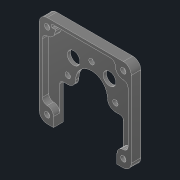
# Autodesk Inventor part: base47
Saved by Autodesk Inventor 2022 (Build 260153000, 153)
## iProperties
Created: 2021-09-10
Part Number: base47
Material: ABS プラスチック
Document SubType Name: Modeling
Designer: Yuta Kage
Density: 1.06 g/cm^3
Appearance: 滑らか - 黒
Author: Yuta Kage
Autodesk Inventor part; units mm, degrees
ref_plane "YZ Plane" through (0, 0, 0) normal (1, 0, 0) x (0, 1, 0)
ref_plane "XZ Plane" through (0, 0, 0) normal (0, 1, 0) x (-1, 0, 0)
ref_plane "XY Plane" through (0, 0, 0) normal (0, 0, 1) x (1, 0, 0)
sketch "スケッチ1" plane through (0, 0, 0) normal (0, 0, 1) x (1, 0, 0)
  line L0 (-29, -29) -> (29, -29)
  line L1 (29, -29) -> (29, 29)
  line L2 (29, 29) -> (-29, 29)
  line L3 (-29, 29) -> (-29, -29)
  line L4 (-29, -29) -> (29, 29) construction
  line L5 (29, -29) -> (-29, 29) construction
  point P0 (0, 0)
  dimension "d0" = 58
  dimension "d1" = 58
  constraints: 12 end point, 2 midpoint, 2 parallel, 1 horizontal, 1 perpendicular
  measures "d0" distance of L2.end L1.end
  measures "d1" distance of L1.end L0.end
extrude "押し出し1" add sketch "スケッチ1" along normal blind 6
fillet "フィレット1" radius 5 4 edges at (-29, 29, 3) (29, 29, 3) (29, -29, 3) (-29, -29, 3)
sketch "スケッチ4" plane through (0, 0, 6) normal (0, 0, 1) x (1, 0, 0)
  arc A0 (-29, -24) -> (-24, -29) centre (-24, -24) ccw projected
  line L0 (-24, -29) -> (24, -29) projected
  arc A1 (24, -29) -> (29, -24) centre (24, -24) ccw projected
  line L1 (29, -24) -> (29, 24) projected
  arc A2 (29, 24) -> (24, 29) centre (24, 24) ccw projected
  line L2 (24, 29) -> (-24, 29) projected
  arc A3 (-24, 29) -> (-29, 24) centre (-24, 24) ccw projected
  line L3 (-29, 24) -> (-29, -24) projected
  line L4 (-27, -27) -> (27, -27)
  line L5 (27, -27) -> (27, 27)
  line L6 (27, 27) -> (-27, 27)
  line L7 (-27, 27) -> (-27, -27)
  line L8 (-27, -27) -> (27, 27) construction
  line L9 (27, -27) -> (-27, 27) construction
  line L10 (-24, -24) -> (24, -24) construction
  line L11 (24, -24) -> (24, 24) construction
  line L12 (24, 24) -> (-24, 24) construction
  line L13 (-24, 24) -> (-24, -24) construction
  line L14 (-24, -24) -> (24, 24) construction
  line L15 (24, -24) -> (-24, 24) construction
  line L16 (24, 29) -> (-24, 29) projected
  circle A4 centre (-24, 24) radius 5
  circle A5 centre (24, 24) radius 5
  arc A6 (24, -29) -> (29, -24) centre (24, -24) ccw projected
  circle A7 centre (24, -24) radius 5
  line L17 (-24, -29) -> (24, -29) projected
  circle A8 centre (-24, -24) radius 5
  line L18 (-29, 29) -> (-19, 29)
  line L19 (-19, 29) -> (-19, 19)
  line L20 (-19, 19) -> (-29, 19)
  line L21 (-29, 19) -> (-29, 29)
  line L22 (-29, 29) -> (-19, 19) construction
  line L23 (-19, 29) -> (-29, 19) construction
  line L24 (29, 29) -> (19, 29)
  line L25 (19, 29) -> (19, 19)
  line L26 (19, 19) -> (29, 19)
  line L27 (29, 19) -> (29, 29)
  line L28 (29, 29) -> (19, 19) construction
  line L29 (19, 29) -> (29, 19) construction
  line L30 (29, -29) -> (19, -29)
  line L31 (19, -29) -> (19, -19)
  line L32 (19, -19) -> (29, -19)
  line L33 (29, -19) -> (29, -29)
  line L34 (29, -29) -> (19, -19) construction
  line L35 (19, -29) -> (29, -19) construction
  line L36 (-29, -29) -> (-19, -29)
  line L37 (-19, -29) -> (-19, -19)
  line L38 (-19, -19) -> (-29, -19)
  line L39 (-29, -19) -> (-29, -29)
  line L40 (-29, -29) -> (-19, -19) construction
  line L41 (-19, -29) -> (-29, -19) construction
  point P0 (0, 0)
  point P1 (-20, -27)
  point P2 (20, -27)
  point P3 (27, -20)
  point P4 (27, 20)
  point P5 (20, 27)
  point P6 (-20, 27)
  point P7 (-27, 20)
  point P8 (-27, -20)
  point P9 (-19, -24)
  point P10 (-19, -27)
  point P11 (19, -27)
  point P12 (19, -24)
  point P13 (24, -19)
  point P14 (27, -19)
  point P15 (27, 19)
  point P16 (24, 19)
  point P17 (19, 24)
  point P18 (19, 27)
  point P19 (-19, 27)
  point P20 (-19, 24)
  point P21 (-24, 19)
  point P22 (-27, 19)
  point P23 (-27, -19)
  point P24 (-24, -19)
  dimension "d77" = 54
  dimension "d78" = 54
  dimension "d79" = 48
  dimension "d80" = 48
  dimension "d81" = 10
  dimension "d82" = 10
  dimension "d83" = 10
  dimension "d84" = 10
  dimension "d85" = 10
  dimension "d86" = 10
  dimension "d87" = 10
  dimension "d88" = 10
  dimension "d89" = 10
  dimension "d90" = 10
  dimension "d91" = 10
  dimension "d92" = 10
  constraints: 72 end point, 13 midpoint, 12 parallel, 6 horizontal, 6 perpendicular, 4 centre point, 4 coincident
  measures "d77" distance of L6.end L5.end
  measures "d78" distance of L5.end L4.end
  measures "d79" distance of L12.end L11.end
  measures "d80" distance of L11.end L10.end
  measures "d81" distance of L19.end L20.end
  measures "d82" distance of L18.end L19.end
  measures "d83" distance of L26.end L25.end
  measures "d84" distance of L25.end L24.end
  measures "d85" distance of L31.end L32.end
  measures "d86" distance of L30.end L31.end
  measures "d87" distance of L38.end L37.end
  measures "d88" distance of L37.end L36.end
  measures "d89" diameter of A4
  measures "d90" diameter of A5
  measures "d91" diameter of A8
  measures "d92" diameter of A7
extrude "押し出し2" cut sketch "スケッチ4" against normal blind 4 contours L7 L20 L19 L6 L25 L26 L5 L32 L31 L4 L37 L38
sketch "スケッチ5" plane through (0, 0, 2) normal (0, 0, 1) x (1, 0, 0)
  circle A0 centre (0, 0) radius 16
  point P0 (-11.3137, 11.3137)
  point P1 (-11.3137, -11.3137)
  point P2 (11.3137, -11.3137)
  point P3 (11.3137, 11.3137)
  dimension "d18" = 32
  dimension "d21" = 360
  dimension "d58" = 0
  constraints: 1 coincident, 8 other
  measures "d58" vertical distance of point (11.314, 11.314) point (-11.314, 11.314)
hole "穴2" at (-11.3137, 11.3137, 2) at (-11.3137, -11.3137, 2) at (11.3137, -11.3137, 2) at (11.3137, 11.3137, 2) direction (0, 0, -1) diameter 4.5 depth 11.8 tip angle 118 counterbore diameter 8 counterbore depth 4 clearance for "Socket Head Cap Screw" size "M4" standard "Ansi Metric M Profile"
sketch "スケッチ6" plane through (0, 0, 2) normal (0, 0, 1) x (1, 0, 0)
  circle A0 centre (0, 0) radius 15
  point P0 (0, 15)
  point P1 (-15, 0)
  point P2 (0, -15)
  point P3 (15, 0)
  dimension "d30" = 30
  dimension "d33" = 360
  dimension "d59" = 0
  constraints: 1 coincident, 1 vertical alignment, 7 other
  measures "d59" horizontal distance of point (0, -15) point (0, 15)
hole "穴3" at (15, 0, 2) at (0, 15, 2) at (-15, 0, 2) direction (0, 0, -1) diameter 3.4 depth 11.8 tip angle 118 clearance for "Socket Head Cap Screw" size "M3" standard "Ansi Metric M Profile"
fillet "フィレット5" radius 3 8 edges at (-27, 19, 4) (-19, 27, 4) (19, 27, 4) (27, 19, 4) (27, -19, 4) (19, -27, 4) (-19, -27, 4) (-27, -19, 4)
sketch "スケッチ7" plane through (0, 0, 2) normal (0, 0, 1) x (1, 0, 0)
  circle A0 centre (0, 0) radius 10
  dimension "d42" = 20
  constraints: 1 centre point, 1 coincident
  measures "d42" diameter of A0
extrude "押し出し3" cut sketch "スケッチ7" against normal through all
sketch "スケッチ8" plane through (0, 0, 6) normal (0, 0, 1) x (1, 0, 0)
  line L0 (24, -24) -> (-24, -24)
  line L1 (-24, -24) -> (-24, 24)
  line L2 (-24, 24) -> (24, 24)
  line L3 (24, 24) -> (24, -24)
  line L4 (24, -24) -> (-24, 24) construction
  line L5 (-24, -24) -> (24, 24) construction
  point P0 (0, 0)
  dimension "d45" = 48
  dimension "d46" = 48
  constraints: 12 end point, 2 midpoint, 2 parallel, 1 horizontal, 1 perpendicular
  measures "d45" distance of L1.end L2.end
  measures "d46" distance of L0.end L1.end
hole "穴4" at (-24, 24, 6) at (-24, -24, 6) at (24, -24, 6) at (24, 24, 6) direction (0, 0, -1) diameter 3.4 depth 6 tip angle 118 clearance for "Flat Head Machine Screw" size "M3" standard "Ansi Metric M Profile"
sketch "スケッチ9" plane through (0, 0, 6) normal (0, 0, 1) x (1, 0, 0)
  line L0 (-20, -29) -> (20, -29)
  line L1 (20, -29) -> (20, -5)
  line L2 (20, -5) -> (-20, -5)
  line L3 (-20, -5) -> (-20, -29)
  line L4 (-20, -29) -> (20, -5) construction
  line L5 (20, -29) -> (-20, -5) construction
  line L6 (-24, -29) -> (24, -29) projected
  circle A0 centre (11.3137, -11.3137) radius 4 projected
  line L7 (10, 5) -> (-10, 5)
  line L8 (-10, 5) -> (-10, -5)
  line L9 (-10, -5) -> (10, -5)
  line L10 (10, -5) -> (10, 5)
  line L11 (10, 5) -> (-10, -5) construction
  line L12 (-10, 5) -> (10, -5) construction
  circle A1 centre (0, 0) radius 10 projected
  line L13 (-10, 0) -> (10, 0)
  point P0 (0, -17)
  point P1 (0, -17)
  point P2 (8.6603, -5)
  point P3 (-8.6603, -5)
  point P4 (-15, 0)
  dimension "d54" = 40
  dimension "d64" = 5
  constraints: 26 end point, 7 midpoint, 4 parallel, 2 horizontal, 2 perpendicular, 2 point on circle, 2 point on line, 1 tangent, 1 vertical alignment
  measures "d54" distance of L1.end L2.end
  measures "d64" distance from line of point (-15, 0) L2
extrude "押し出し4" cut sketch "スケッチ9" against normal through all contours L3 L2 A1 L1 L0 | L8 A1 L2 | L2 A1 L10 | L2 A1 | A0
fillet "フィレット7" radius 5 2 edges at (-10, -5, 1) (10, -5, 1)
fillet "フィレット8" radius 2 2 edges at (-20, -5, 1) (20, -5, 1)
sketch "スケッチ11" plane through (0, 0, 0) normal (0, 0, -1) x (-1, 0, 0)
  circle A0 centre (24, 24) radius 1.7 projected
  circle A1 centre (24, -24) radius 1.7 projected
  circle A2 centre (-24, 24) radius 1.7 projected
  circle A3 centre (-24, -24) radius 1.7 projected
  line L0 (26.8, 25.6166) -> (26.8, 22.3834)
  line L1 (26.8, 22.3834) -> (24, 20.7668)
  line L2 (24, 20.7668) -> (21.2, 22.3834)
  line L3 (21.2, 22.3834) -> (21.2, 25.6166)
  line L4 (21.2, 25.6166) -> (24, 27.2332)
  line L5 (24, 27.2332) -> (26.8, 25.6166)
  line L6 (-24, 29) -> (24, 29) projected
  line L7 (21.2, -25.6166) -> (21.2, -22.3834)
  line L8 (21.2, -22.3834) -> (24, -20.7668)
  line L9 (24, -20.7668) -> (26.8, -22.3834)
  line L10 (26.8, -22.3834) -> (26.8, -25.6166)
  line L11 (26.8, -25.6166) -> (24, -27.2332)
  line L12 (24, -27.2332) -> (21.2, -25.6166)
  line L13 (-21.2, 25.6166) -> (-21.2, 22.3834)
  line L14 (-21.2, 22.3834) -> (-24, 20.7668)
  line L15 (-24, 20.7668) -> (-26.8, 22.3834)
  line L16 (-26.8, 22.3834) -> (-26.8, 25.6166)
  line L17 (-26.8, 25.6166) -> (-24, 27.2332)
  line L18 (-24, 27.2332) -> (-21.2, 25.6166)
  line L19 (24, -29) -> (20, -29) projected
  line L20 (-21.2, -22.3834) -> (-21.2, -25.6166)
  line L21 (-21.2, -25.6166) -> (-24, -27.2332)
  line L22 (-24, -27.2332) -> (-26.8, -25.6166)
  line L23 (-26.8, -25.6166) -> (-26.8, -22.3834)
  line L24 (-26.8, -22.3834) -> (-24, -20.7668)
  line L25 (-24, -20.7668) -> (-21.2, -22.3834)
  arc A4 (-29, -24) -> (-24, -29) centre (-24, -24) ccw projected
  line L26 (-20, -29) -> (-24, -29) projected
  line L27 (-29, -24) -> (-24, -29)
  point P0 (0, 0)
  point P1 (-25.8144, -26.1856)
  point P2 (-26.8, -25.2)
  dimension "d31" = 4
  dimension "d67" = 5.6
  dimension "d68" = 30
  dimension "d69" = 5.6
  dimension "d70" = 30
  dimension "d71" = 30
  dimension "d72" = 5.6
  dimension "d73" = 15
  dimension "d74" = 5.6
  constraints: 50 end point, 4 coincident, 52 other
  measures "d67" distance between parallel lines of L3 L0
  measures "d68" angle of L6 L5
  measures "d69" distance between parallel lines of L14 L17
  measures "d70" angle of L6 L17
  measures "d71" angle of L19 L11
  measures "d72" distance between parallel lines of L12 L9
  measures "d73" angle of L22 L27
  measures "d74" distance between parallel lines of L24 L21
extrude "押し出し5" cut sketch "スケッチ11" against normal blind 4 contours A0 | A1 | A2 | A3 | L0 L1 L2 L3 L4 L5 | L7 L8 L9 L10 L11 L12 | L13 L14 L15 L16 L17 L18 | L20 L21 L22 L23 L24 L25
sketch "スケッチ12" plane through (0, 0, 6) normal (0, 0, 1) x (1, 0, 0)
  line L0 (-21, 25) -> (-3.9723, 25)
  line L1 (-3.9723, 25) -> (-3.9723, 27)
  line L2 (-3.9723, 27) -> (-21, 27)
  line L3 (-21, 27) -> (-21, 25)
  line L4 (-21, 25) -> (-3.9723, 27) construction
  line L5 (-3.9723, 25) -> (-21, 27) construction
  line L6 (24, 29) -> (-24, 29) projected
  line L7 (29, -24) -> (29, 24) projected
  line L8 (-29, 24) -> (-29, -24) projected
  line L9 (-19, 19) -> (-19, 24) projected
  line L10 (-19, 24) -> (-17.5063, 24)
  line L11 (-17.5063, 24) -> (-17.5063, 25)
  line L12 (-17.5063, 25) -> (-19, 25)
  line L13 (-19, 25) -> (-19, 24)
  point P0 (0, 0)
  point P1 (-12.4862, 26)
  point P2 (29, -19)
  dimension "d93" = 3
  dimension "d98" = 8
  dimension "d99" = 2
  constraints: 20 end point, 4 parallel, 2 horizontal, 2 midpoint, 2 perpendicular, 1 point on line
  measures "d93" distance from line of L6 point (-12.486, 26)
  measures "d98" distance between parallel lines of L8 L3
  measures "d99" distance of L2.end L0.start
extrude "押し出し6" cut sketch "スケッチ12" against normal up to surface (4 mm away)
fillet "フィレット9" radius 4 2 edges at (-20, -19, 4) (20, -19, 4)
fillet "フィレット10" radius 5 2 edges at (19, 19, 4) (-19, 19, 4)
equation "\"d0\" = d1"
equation "\"d78\" = d77"
equation "\"d81\" = d89"
equation "\"d82\" = d89"
equation "\"d83\" = d90"
equation "\"d84\" = d90"
equation "\"d85\" = d92"
equation "\"d86\" = d92"
equation "\"d87\" = d91"
equation "\"d88\" = d91"
equation "\"d89\" = d90"
equation "\"d91\" = d89"
equation "\"d92\" = d91"
